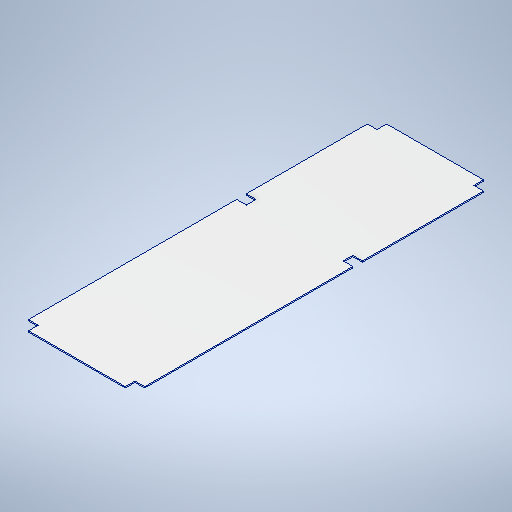
# Autodesk Inventor part: benchtop
Saved by Autodesk Inventor 2025 (Build 290162010, 162A)
## iProperties
Created: 2024-06-14
Part Number: benchtop
Material: Aluminum 6061
Document SubType Name: Modeling
Designer: Alan Thomas
Mass: 9460.8 g
Surface Area: 14220 cm^2
Volume: 3504 cm^3
Density: 2.7 g/cm^3
Appearance: Aluminum - Flat
Author: Alan Thomas
Autodesk Inventor part; units mm, degrees
ref_plane "YZ Plane" through (0, 0, 0) normal (1, 0, 0) x (0, 1, 0)
ref_plane "XZ Plane" through (0, 0, 0) normal (0, 1, 0) x (-1, 0, 0)
ref_plane "XY Plane" through (0, 0, 0) normal (0, 0, 1) x (1, 0, 0)
sketch "Sketch1" plane through (0, 0, 0) normal (0, 1, 0) x (-1, 0, 0)
  line L0 (0, 0) -> (480, 0)
  line L1 (480, 0) -> (480, -1480)
  line L2 (480, -1480) -> (0, -1480)
  line L3 (0, -1480) -> (0, 0)
  dimension "d0" = 480
  dimension "d1" = 1480
  constraints: 8 end point, 2 parallel, 1 horizontal, 1 perpendicular
  measures "d0" distance of L1.end L2.end
  measures "d1" distance of L0.end L1.end
extrude "Extrusion1" add sketch "Sketch1" along normal blind 5
sketch "Sketch2" plane through (0, 5, 0) normal (0, 1, 0) x (1, 0, 0)
  line L0 (0, 0) -> (-40, 0)
  line L1 (-40, 0) -> (-40, 40)
  line L2 (-40, 40) -> (0, 40)
  line L3 (0, 40) -> (0, 0)
  dimension "d4" = 40
  dimension "d5" = 40
  constraints: 8 end point, 2 parallel, 1 horizontal, 1 perpendicular
  measures "d4" distance of L1.end L2.end
  measures "d5" distance of L0.end L1.end
extrude "Extrusion2" cut sketch "Sketch2" against normal blind 10
sketch "Sketch3" plane through (0, 5, 0) normal (0, 1, 0) x (1, 0, 0)
  line L0 (-480, 0) -> (-440, 0)
  line L1 (-440, 0) -> (-440, 40)
  line L2 (-440, 40) -> (-480, 40)
  line L3 (-480, 40) -> (-480, 0)
  point P0 (0, 0)
  dimension "d8" = 40
  dimension "d9" = 40
  constraints: 8 end point, 2 parallel, 1 horizontal, 1 perpendicular
  measures "d8" distance of L2.end L1.end
  measures "d9" distance of L1.end L0.end
extrude "Extrusion3" cut sketch "Sketch3" against normal blind 10
sketch "Sketch4" plane through (0, 5, 0) normal (0, 1, 0) x (1, 0, 0)
  line L0 (0, 1480) -> (-480, 1480) projected
  line L1 (0, 1480) -> (-40, 1480)
  line L2 (-40, 1480) -> (-40, 1440)
  line L3 (-40, 1440) -> (0, 1440)
  line L4 (0, 1440) -> (0, 1480)
  point P0 (0, 0)
  dimension "d12" = 40
  dimension "d13" = 40
  constraints: 8 end point, 2 parallel, 1 horizontal, 1 perpendicular
  measures "d12" distance of L3.end L2.end
  measures "d13" distance of L2.end L1.end
extrude "Extrusion4" cut sketch "Sketch4" against normal blind 10
sketch "Sketch5" plane through (0, 5, 0) normal (0, 1, 0) x (1, 0, 0)
  line L0 (-40, 1480) -> (-480, 1480) projected
  line L1 (-480, 1480) -> (-440, 1480)
  line L2 (-440, 1480) -> (-440, 1440)
  line L3 (-440, 1440) -> (-480, 1440)
  line L4 (-480, 1440) -> (-480, 1480)
  point P0 (0, 0)
  dimension "d16" = 40
  dimension "d17" = 40
  constraints: 8 end point, 2 parallel, 1 horizontal, 1 perpendicular
  measures "d16" distance of L2.end L3.end
  measures "d17" distance of L1.end L2.end
extrude "Extrusion5" cut sketch "Sketch5" against normal blind 10
sketch "Sketch7" plane through (0, 5, 0) normal (0, 1, 0) x (1, 0, 0)
  line L0 (0, 40) -> (0, 1440) projected
  line L1 (0, 940) -> (-40, 940)
  line L2 (-40, 940) -> (-40, 900)
  line L3 (-40, 900) -> (0, 900)
  line L4 (0, 900) -> (0, 940)
  point P0 (0, 0)
  point P1 (0, 760)
  point P2 (0, 900)
  dimension "d24" = 40
  dimension "d25" = 40
  constraints: 8 end point, 2 parallel, 1 horizontal, 1 perpendicular, 1 point on line
  measures "d24" distance of L3.end L2.end
  measures "d25" distance of L2.end L1.end
extrude "Extrusion7" cut sketch "Sketch7" against normal blind 10
sketch "Sketch8" plane through (0, 5, 0) normal (0, 1, 0) x (1, 0, 0)
  line L0 (-480, 1440) -> (-480, 40) projected
  line L1 (-480, 900) -> (-440, 900)
  line L2 (-440, 900) -> (-440, 940)
  line L3 (-440, 940) -> (-480, 940)
  line L4 (-480, 940) -> (-480, 900)
  point P0 (0, 0)
  dimension "d28" = 40
  dimension "d29" = 40
  constraints: 8 end point, 2 parallel, 1 horizontal, 1 perpendicular, 1 point on line
  measures "d28" distance of L3.end L2.end
  measures "d29" distance of L2.end L1.end
extrude "Extrusion8" cut sketch "Sketch8" against normal blind 10
body "Solid1"
